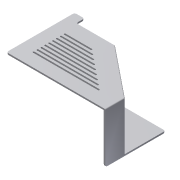
# Autodesk Inventor part: ControlMockup
Saved by Autodesk Inventor 2014 (Build 180170000, 170)
## iProperties
Created: 2014-08-14
Part Number: ControlMockup
Material: Generic
Document SubType Name: Modeling
Designer: Peele
Density: 1 g/cm^3
Appearance: White
Author: Peele
Autodesk Inventor part; units mm, degrees
ref_plane "YZ Plane" through (0, 0, 0) normal (1, 0, 0) x (0, 1, 0)
ref_plane "XZ Plane" through (0, 0, 0) normal (0, 1, 0) x (-1, 0, 0)
ref_plane "XY Plane" through (0, 0, 0) normal (0, 0, 1) x (1, 0, 0)
sketch "Sketch1" plane through (0, 0, 0) normal (0, 0, 1) x (1, 0, 0)
  line L0 (0, 175) -> (0, 0)
  line L1 (0, 0) -> (254, 0)
  line L2 (254, 0) -> (254, 50)
  line L3 (254, 50) -> (125, 154)
  line L4 (125, 154) -> (25, 154)
  line L5 (25, 154) -> (25, 175)
  line L6 (25, 175) -> (0, 175)
  dimension "d0" = 175
  dimension "d1" = 254
  dimension "d2" = 25
  dimension "d3" = 50
  dimension "d4" = 21
  dimension "d5" = 100
  constraints: 14 end point, 4 parallel, 1 perpendicular, 1 vertical
  measures "d0" distance of L0.start L0.end
  measures "d1" distance of L0.end L1.end
  measures "d2" distance of L5.end L0.start
  measures "d3" distance of L1.end L2.end
  measures "d4" distance of L4.end L5.end
  measures "d5" distance of L3.end L4.end
extrude "Extrusion1" add sketch "Sketch1" along normal blind 4
sketch "Sketch2" plane through (0, 0, 0) normal (0, 0, -1) x (-1, 0, 0)
  line L0 (-25, 154) -> (-125, 154) projected
  line L1 (-125, 154) -> (-254, 50) projected
  line L2 (-254, 50) -> (-254, 0) projected
  line L3 (-254, 0) -> (0, 0) projected
  line L4 (-25, 154) -> (-125, 154)
  line L5 (-125, 154) -> (-254, 50)
  line L6 (-254, 50) -> (-254, 0)
  line L7 (-254, 0) -> (-250, 0)
  line L8 (-250, 0) -> (-250, 48.0868)
  line L9 (-250, 48.0868) -> (-123.5884, 150)
  line L10 (-123.5884, 150) -> (-25, 150)
  line L11 (-25, 150) -> (-25, 154)
  dimension "d8" = 4
  dimension "d9" = 4
  dimension "d10" = 4
  constraints: 16 end point, 3 collinear, 2 parallel, 2 perpendicular, 1 point on line
  measures "d8" distance between parallel lines of L4 L10
  measures "d9" distance between parallel lines of L1 L9
  measures "d10" distance between parallel lines of L2 L8
extrude "Extrusion2" add sketch "Sketch2" along normal blind 125
sketch "Sketch3" plane through (0, 0, -125) normal (0, 0, -1) x (-1, 0, 0)
  line L0 (-125, 154) -> (-254, 50) projected
  line L1 (-123.5884, 150) -> (-25, 150) projected
  line L2 (-25, 150) -> (-25, 154) projected
  line L3 (-254, 50) -> (-254, 154)
  line L4 (-254, 154) -> (-125, 154)
  line L5 (-254, 50) -> (-125, 154)
  point P0 (0, 0)
  constraints: 6 end point, 2 parallel, 1 collinear
extrude "Extrusion3" add sketch "Sketch3" against normal blind 4
fillet "Fillet1" radius 5 7 edges at (0, 0, 2) (25, 154, 2) (25, 175, 2) (0, 175, 2) (254, 154, -123) (25, 152, -125) (252, 0, -125)
fillet "Fillet2" radius 2 4 edges at (189.5, 102, 4) (254, 50, -58.5) (254, 25, 4) (125, 154, -58.5)
sketch "Sketch4" plane through (0, 0, 4) normal (0, 0, 1) x (1, 0, 0)
  line L0 (121.8134, 154) -> (252, 49.0434) projected
  line L1 (0, 170) -> (0, 5) projected
  line L2 (5, 0) -> (252, 0) projected
  line L3 (252, 49.0434) -> (252, 0) projected
  line L4 (35, 35) -> (202, 35) construction
  line L5 (35, 33) -> (202, 33)
  line L6 (202, 37) -> (35, 37)
  arc A0 (35, 37) -> (35, 33) centre (35, 35) ccw
  arc A1 (202, 33) -> (202, 37) centre (202, 35) ccw
  line L7 (35, 45) -> (189.5962, 45) construction
  line L8 (35, 43) -> (189.5962, 43)
  line L9 (189.5962, 47) -> (35, 47)
  arc A2 (35, 47) -> (35, 43) centre (35, 45) ccw
  arc A3 (189.5962, 43) -> (189.5962, 47) centre (189.5962, 45) ccw
  line L10 (35, 55) -> (177.1923, 55) construction
  line L11 (35, 53) -> (177.1923, 53)
  line L12 (177.1923, 57) -> (35, 57)
  arc A4 (35, 57) -> (35, 53) centre (35, 55) ccw
  arc A5 (177.1923, 53) -> (177.1923, 57) centre (177.1923, 55) ccw
  line L13 (35, 65) -> (164.7885, 65) construction
  line L14 (35, 63) -> (164.7885, 63)
  line L15 (164.7885, 67) -> (35, 67)
  arc A6 (35, 67) -> (35, 63) centre (35, 65) ccw
  arc A7 (164.7885, 63) -> (164.7885, 67) centre (164.7885, 65) ccw
  line L16 (35, 75) -> (152.3846, 75) construction
  line L17 (35, 73) -> (152.3846, 73)
  line L18 (152.3846, 77) -> (35, 77)
  arc A8 (35, 77) -> (35, 73) centre (35, 75) ccw
  arc A9 (152.3846, 73) -> (152.3846, 77) centre (152.3846, 75) ccw
  line L19 (35, 85) -> (139.9808, 85) construction
  line L20 (35, 83) -> (139.9808, 83)
  line L21 (139.9808, 87) -> (35, 87)
  arc A10 (35, 87) -> (35, 83) centre (35, 85) ccw
  arc A11 (139.9808, 83) -> (139.9808, 87) centre (139.9808, 85) ccw
  line L22 (35, 95) -> (127.5769, 95) construction
  line L23 (35, 93) -> (127.5769, 93)
  line L24 (127.5769, 97) -> (35, 97)
  arc A12 (35, 97) -> (35, 93) centre (35, 95) ccw
  arc A13 (127.5769, 93) -> (127.5769, 97) centre (127.5769, 95) ccw
  line L25 (202, 35) -> (71.038, 140.5818) construction
  line L26 (35, 105) -> (115.1731, 105) construction
  line L27 (35, 107) -> (115.1731, 107)
  line L28 (115.1731, 103) -> (35, 103)
  arc A14 (35, 107) -> (35, 103) centre (35, 105) ccw
  arc A15 (115.1731, 103) -> (115.1731, 107) centre (115.1731, 105) ccw
  line L29 (35, 115) -> (102.7692, 115) construction
  line L30 (35, 113) -> (102.7692, 113)
  line L31 (102.7692, 117) -> (35, 117)
  arc A16 (35, 117) -> (35, 113) centre (35, 115) ccw
  arc A17 (102.7692, 113) -> (102.7692, 117) centre (102.7692, 115) ccw
  point P0 (0, 0)
  point P1 (118.5, 35)
  point P2 (112.2981, 45)
  point P3 (106.0962, 55)
  point P4 (99.8942, 65)
  point P5 (93.6923, 75)
  point P6 (87.4904, 85)
  point P7 (81.2885, 95)
  point P8 (75.0865, 105)
  point P9 (68.8846, 115)
  dimension "d17" = 2
  dimension "d18" = 6
  dimension "d19" = 6
  dimension "d20" = 6
  dimension "d21" = 6
  dimension "d22" = 6
  dimension "d23" = 6
  dimension "d24" = 35
  dimension "d25" = 35
  dimension "d26" = 50
  dimension "d27" = 6
  dimension "d28" = 6
  constraints: 72 end point, 36 point on circle, 36 tangent, 18 centre point, 17 parallel, 9 midpoint, 8 equal radius, 8 vertical alignment, 1 perpendicular, 12 other
  measures "d17" radius of A0
  measures "d18" distance between parallel lines of L8 L6
  measures "d19" distance between parallel lines of L11 L9
  measures "d20" distance between parallel lines of L14 L12
  measures "d21" distance between parallel lines of L17 L15
  measures "d22" distance between parallel lines of L20 L18
  measures "d23" distance between parallel lines of L23 L21
  measures "d24" distance between parallel lines of L2 L4
  measures "d25" distance from line of L4.start L1
  measures "d26" distance from line of L4.end L3
  measures "d27" distance between parallel lines of L28 L24
  measures "d28" distance between parallel lines of L30 L27
extrude "Extrusion4" cut sketch "Sketch4" against normal blind 4
equation "\"d9\" = d8"
equation "\"d10\" = d9"
equation "\"d19\" = d18"
equation "\"d20\" = d19"
equation "\"d21\" = d19"
equation "\"d22\" = d21"
equation "\"d23\" = d22"
equation "\"d27\" = d19"
equation "\"d28\" = d21"
body "Solid1"
